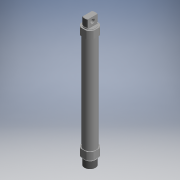
# Autodesk Inventor part: 193993 DSNU-40-300-P---(A----0-ZR)
Saved by Autodesk Inventor 2017.3 (Build 213256000, 256)
## iProperties
Part Number: 193993 DSNU-40-300-P---(A----0-ZR)
Material: Generic
Catalog Web Link: www.cadenas.de
Description: DSNU---(ZR)-Standard cylinder
Vendor: FESTO
Document SubType Name: Modeling
Designer: partserver
Manufacturer: FESTO
Mass: 189.528 g
Surface Area: 1081.04 cm^2
Volume: 189.528 cm^3
Density: 1 g/cm^3
Appearance: PSOLRGB-192-192-192
Category: PARTsolutions
Company: FESTO
Title: 193993 DSNU-40-300-P
Author: Cadenas PARTsolutions
Comments: Standard cylinder
PSOL_IDENT_0: {$CADENAS_DATA\23d-libs\festo\parts\d\dsnu\parts\dsnu_metric_zr.prj},236 {VTYP=3D},{NB=193993 DSNU-4
PSOL_IDENT_1: 0-300-P---(A----0-ZR)},{LINA=193993 DSNU-40-300-P},{NN=DSNU---(ZR)},{DATE=23.06.2020 07:36:16},{GEOM
PSOL_IDENT_2: DATE=06.03.2020 09:03:14},{VERSION=},{LINEID=80},{WBVAR=TNR,HUB,DA,PE,ZD,VS,KA,K8,KP,R8},{WBNUMERIC=
PSOL_IDENT_3: HUB,K8}  {NB=193993 DSNU-40-300-P---(A----0-ZR)},{LINA=193993 DSNU-40-300-P},{KT=DUMMY},{TNR=193993}
PSOL_IDENT_4: ,{TYP=DSNU-40},{DSNU=METRIC},{DE=D},{KDM=40},{HUB=300},{DA=P},{DA1='P','PPV','PPS'},{PE=A},{ZD=-},{V
PSOL_IDENT_5: S=-},{VSALG='-','Q'},{KA=-},{KAALG='-','S2'},{K8=0},{KP=-},{KPALG='-','KP'},{R8=-},{R81='-','R8'},{R
PSOL_IDENT_6: 8H=30.200},{A1=35},{A2=500},{A3=8},{A4=70.5},{AB=38},{AM=24},{B=38},{BB=4},{BE=M38x1,5},{BENDM=38.00
PSOL_IDENT_7: 0},{BEKDM=36.160},{BEP=1.500},{BS=9.0},{B1=54},{B2=13},{B3=38},{B4=12},{B5=32.0},{B6=14},{B7=4},{CD=
PSOL_IDENT_8: 12},{D=46},{D1=38},{D2=16},{D3=41.6},{D4=12.0},{D5=42.0},{D6=50},{D7=38},{EE=G1/4},{EENDM=13.1570},{
PSOL_IDENT_9: EEKDM=11.4450},{EW=18},{F=42},{FF=M5},{FFNDM=5.000},{FFKDM=4.019},{F1=24},{H=48},{H1=7},{KK=M12x1.25
PSOL_IDENT_10: },{KKNDM=12.0000},{KKKDM=9.8530},{KKP=1.250},{K1=M8},{K1NDM=8.000},{K1KDM=6.466},{K2=3.0},{KV=0},{KW=
PSOL_IDENT_11: 10},{L=15},{LH=15.0},{LK=18.0},{L1=153.6},{L2=84.6},{L3=12.0},{L4=30.0},{L5=27},{L6=63},{L7=33},{L8=
PSOL_IDENT_12: 25.0},{L9=29.0},{L10=104.6},{L11=116.6},{L12=77.6},{L13=162.6},{ST=9.0},{SW=13},{T=12},{WH=39},{X=3.
PSOL_IDENT_13: 3},{XC=139.6},{K1KP=56},{K2KP=M8},{K2KPNDM=8.000},{K3KP=18},{K4KP=28.0},{K5KP=89.0},{K6KP=6.8},{K7KP=
PSOL_IDENT_14: 24},{K8KP=36.0},{K9KP=17.0},{K10KP=7.0},{K11KP=20},{K12KP=G1/8},{K12KPNDM=9.728},{K13KP=69},{ZRSTART=
PSOL_IDENT_15: 55},{MHL=45.000},{ZRL=34.6},{C=21.200},{WHX=12.000},{LD1=35.800},{LD2=35.700},{AD1=14.000},{AD2=12.0
PSOL_IDENT_16: 00},{AD3=10.500},{AD4=9.000},{AD5=12.500},{MH1=11.000},{MH2=2.600},{MH3=15.200},{KP1=34.000},{KP2=30
PSOL_IDENT_17: .000},{KP3=24.000},{KP4=25.000},{KP5=45.000},{KPC=22.000},{KPF=3.000},{KPG=22.000},{KPH=83.000},{KPJ=
PSOL_IDENT_18: 23.500},{KPK=17.000},{KPL=4.500},{KPR3=1.000},{KPR=23.000},{KPS=20.500},{MLD1=55.000},{MLD2=48.000},
PSOL_IDENT_19: {MLD3=5.000},{MLL1=16.000},{PPVSTD=18.500},{PPVMH=37.000},{PPVMQ=6.500},{PPVY=10.500},{PPVZ=15.800},
PSOL_IDENT_20: {PPVA=5.000},{PPVB=0.500},{PPVC=0.800},{PPVD=1.000},{PPVE=10.000},{PPVH=16.100},{KL1=76},{SWL=6.500}
PSOL_IDENT_21: ,{K3L=8.400},{ES1=2.500},{ES2=10.500},{KPVERS=0},{HUB1=300},{NUTOFF=8.500},{DIMZJREAR=444.6},{KAVERS=
PSOL_IDENT_22: 0},{VERS=2},{H2=45}
NB: 193993 DSNU-40-300-P---(A----0-ZR)
NN: DSNU---(ZR)
NT: Standard cylinder
NBSYN: $TNR. $TYP.-$HUB1.-$DA.---($PE.$ZD.$VS.$KA.$KP.$K8.$R8.ZR)
LINA: 193993 DSNU-40-300-P
CATALOG: Festo
TNR: 193993
TYP: DSNU-40
DSNU: METRIC
DE: D
KDM: 40
HUB: 300
DA: P
DA1: 'P','PPV','PPS'
PE: A
ZD: -
VS: -
KA: -
K8: 0
KP: -
R8: -
R81: '-','R8'
R8H: 30.2
A1: 35
A2: 500
A3: 8
A4: 70.5
AB: 38
AM: 24
B: 38
BB: 4
BE: M38x1,5
BENDM: 38
BEKDM: 36.16
BEP: 1.5
BS: 9
B1: 54
B2: 13
B3: 38
B4: 12
B5: 32
B6: 14
B7: 4
CD: 12
D: 46
D1: 38
D2: 16
D3: 41.6
D4: 12
D5: 42
D6: 50
D7: 38
EE: G1/4
EENDM: 13.157
EEKDM: 11.445
EW: 18
F: 42
FF: M5
FFNDM: 5
FFKDM: 4.019
F1: 24
H: 48
H1: 7
KK: M12x1.25
KKNDM: 12
KKKDM: 9.853
KKP: 1.25
K1: M8
K1NDM: 8
K1KDM: 6.466
K2: 3
KV: 0
KW: 10
L: 15
LH: 15
LK: 18
L3: 12
L4: 30
L5: 27
L6: 63
L7: 33
L8: 25
L9: 29
L13: 162.6
ST: 9
SW: 13
T: 12
X: 3.3
K1KP: 56
K2KP: M8
K2KPNDM: 8
K3KP: 18
K4KP: 28
K5KP: 89
K6KP: 6.8
K7KP: 24
K8KP: 36
K9KP: 17
K10KP: 7
K11KP: 20
K12KP: G1/8
K12KPNDM: 9.728
K13KP: 69
MHL: 45
C: 21.2
WHX: 12
LD1: 35.8
LD2: 35.7
AD1: 14
AD2: 12
AD3: 10.5
AD4: 9
AD5: 12.5
MH1: 11
MH2: 2.6
MH3: 15.2
KP1: 34
KP2: 30
KP3: 24
KP4: 25
KP5: 45
KPC: 22
KPF: 3
KPG: 22
KPH: 83
KPJ: 23.5
KPK: 17
KPL: 4.5
KPR3: 1
KPR: 23
KPS: 20.5
MLD1: 55
MLD2: 48
MLD3: 5
MLL1: 16
PPVSTD: 18.5
PPVMH: 37
PPVMQ: 6.5
PPVY: 10.5
PPVZ: 15.8
PPVA: 5
PPVB: 0.5
PPVC: 0.8
PPVD: 1
PPVE: 10
PPVH: 16.1
SWL: 6.5
K3L: 8.4
ES1: 2.5
ES2: 10.5
NUTOFF: 8.5
H2: 45
SUPPLIER: FESTO
ARTICLENO: 193993 DSNU-40-300-P---(A----0-ZR)
BOMINFO: 193993 DSNU-40-300-P
CREATOR: CADENAS GmbH
Autodesk Inventor part; units mm, degrees
sketch "Sketch_12" plane through (0, 0, 0) normal (1, 0, 0) x (0, 1, 0)
  line L0 (0, -444.6) -> (0, 0)
  line L1 (0, 0) -> (18.08, 0)
  line L2 (18.08, 0) -> (19, -0.92)
  line L3 (19, -0.92) -> (19, -23.95)
  line L4 (19, -23.95) -> (18.0843, -24.8657)
  arc A0 (18.0843, -24.8657) -> (17.85, -25.4314) centre (18.65, -25.4314) ccw
  line L5 (17.85, -25.4314) -> (17.85, -26.2)
  arc A1 (17.85, -26.2) -> (18.65, -27) centre (18.65, -26.2) ccw
  line L6 (18.65, -27) -> (19, -27)
  line L7 (19, -27) -> (19, -30.1)
  line L8 (19, -30.1) -> (24.5, -30.1)
  line L9 (24.5, -30.1) -> (24.5, -55.05)
  line L10 (24.5, -55.05) -> (20.8, -55.05)
  line L11 (20.8, -55.05) -> (20.8, -389.55)
  line L12 (20.8, -389.55) -> (24.5, -389.55)
  line L13 (24.5, -389.55) -> (24.5, -414.5)
  line L14 (24.5, -414.5) -> (19, -414.5)
  line L15 (19, -414.5) -> (19, -417.6)
  line L16 (19, -417.6) -> (18.65, -417.6)
  arc A2 (18.65, -417.6) -> (17.85, -418.4) centre (18.65, -418.4) ccw
  line L17 (17.85, -418.4) -> (17.85, -419.1686)
  arc A3 (17.85, -419.1686) -> (18.0843, -419.7343) centre (18.65, -419.1686) ccw
  line L18 (18.0843, -419.7343) -> (19, -420.65)
  line L19 (19, -420.65) -> (19, -443.68)
  line L20 (19, -443.68) -> (18.08, -444.6)
  line L21 (18.08, -444.6) -> (0, -444.6)
  line L22 (0, -444.6) -> (0, 0)
  constraints: 46 end point, 8 point on circle, 4 centre point
revolve "Revolution1" add sketch "Sketch_12" angle 360 about axis through (0, 0, -444.6) along (0, 0, -1)
thread "Thread1" size "M38x1.5" class "6g" standard "ISO Metric profile" full length
thread "Thread2" size "M38x1.5" class "6g" standard "ISO Metric profile" full length
sketch "Sketch_1" plane through (0, 0, 0) normal (0, 0, 1) x (1, 0, 0)
  line L0 (-45, 45) -> (-45, -45)
  line L1 (-45, -45) -> (45, -45)
  line L2 (45, -45) -> (45, 45)
  line L3 (45, 45) -> (-45, 45)
  line L4 (-22.5, 22.5) -> (-22.5, -22.5)
  line L5 (-22.5, -22.5) -> (22.5, -22.5)
  line L6 (22.5, -22.5) -> (22.5, 22.5)
  line L7 (22.5, 22.5) -> (-22.5, 22.5)
  constraints: 16 end point
extrude "Extrusion1" cut sketch "Sketch_1" against normal blind 453.6
sketch "Sketch_124" plane through (0, 0, 0) normal (0, 1, 0) x (-1, 0, 0)
  line L0 (46, -415.6) -> (9, -415.6)
  line L1 (9, -415.6) -> (9, -444.6)
  line L2 (9, -444.6) -> (-9, -444.6)
  line L3 (-9, -444.6) -> (-9, -415.6)
  line L4 (-9, -415.6) -> (-46, -415.6)
  line L5 (-46, -415.6) -> (-46, -449.6)
  line L6 (-46, -449.6) -> (46, -449.6)
  line L7 (46, -449.6) -> (46, -415.6)
  constraints: 16 end point
extrude "Extrusion2" cut sketch "Sketch_124" along normal mid plane 46
sketch "Sketch_3" plane through (0, 0, -430.6) normal (0, 0, 1) x (1, 0, 0)
  line L0 (9, 0) -> (-9, 0)
  line L1 (-9, 0) -> (-9, 7.5774)
  line L2 (-9, 7.5774) -> (-8, 7)
  line L3 (-8, 7) -> (-7.5, 7)
  line L4 (-7.5, 7) -> (-7.5, 6)
  line L5 (-7.5, 6) -> (7.5, 6)
  line L6 (7.5, 6) -> (7.5, 7)
  line L7 (7.5, 7) -> (8, 7)
  line L8 (8, 7) -> (9, 7.5774)
  line L9 (9, 7.5774) -> (9, 0)
  line L10 (9, 0) -> (-9, 0)
  constraints: 22 end point
revolve "Revolution2" cut sketch "Sketch_3" angle 360 about axis through (9, 0, -430.6) along (1, 0, 0)
sketch "Sketch5" plane through (-9.6954, 22.5, -30.1) normal (0, 1, 0) x (1, 0, 0)
  point P0 (9.6954, 12)
hole "Hole1" at (0, 22.5, -42.1) direction (0, -1, 0) diameter 11.445 depth 22.5 countersink diameter 13.157 countersink angle 90 thread size "G13.157x1.337" designation "G 1/4" standard "ISO Pipe Threads"
sketch "Sketch6" plane through (-9.6954, 22.5, -389.55) normal (0, 1, 0) x (1, 0, 0)
  point P0 (9.6954, 12.95)
hole "Hole2" at (0, 22.5, -402.5) direction (0, -1, 0) diameter 11.445 depth 10.5 tip angle 120 countersink diameter 13.157 countersink angle 90 thread size "G13.157x1.337" designation "G 1/4" standard "ISO Pipe Threads"
sketch "Sketch_129" plane through (0, 0, 0) normal (1, 0, 0) x (0, 1, 0)
  line L0 (0, -377) -> (0, 9)
  line L1 (0, 9) -> (8, 9)
  line L2 (8, 9) -> (8, -67)
  line L3 (8, -67) -> (20, -67)
  line L4 (20, -67) -> (20, -377)
  line L5 (20, -377) -> (0, -377)
  line L6 (0, -377) -> (0, 9)
  constraints: 14 end point
revolve "Revolution3" cut sketch "Sketch_129" angle 360 about axis through (0, 0, -377) along (0, 0, -1)
ref_plane "FDT_FRONT_XY" through (0, 0, -30.1) normal (0, 0, -1) x (1, 0, 0)
ref_plane "FDT_FRONT_YZ" through (0, 0, -30.1) normal (1, 0, 0) x (0, -1, 0)
ref_plane "FDT_FRONT_ZX" through (0, 0, -30.1) normal (0, -1, 0) x (0, 0, -1)
ref_plane "FDT_QSFRONT_XY" through (0, 22.5, -42.1) normal (0, 1, 0) x (0, 0, 1)
ref_plane "FDT_QSFRONT_YZ" through (0, 22.5, -42.1) normal (0, 0, 1) x (1, 0, 0)
ref_plane "FDT_QSFRONT_ZX" through (0, 22.5, -42.1) normal (1, 0, 0) x (0, 1, 0)
ref_plane "FDT_QSREAR_XY" through (0, 22.5, -402.5) normal (0, 1, 0) x (0, 0, 1)
ref_plane "FDT_QSREAR_YZ" through (0, 22.5, -402.5) normal (0, 0, 1) x (1, 0, 0)
ref_plane "FDT_QSREAR_ZX" through (0, 22.5, -402.5) normal (1, 0, 0) x (0, 1, 0)
ref_plane "FDT_REAR_XY" through (0, 0, -414.5) normal (0, 0, 1) x (1, 0, 0)
ref_plane "FDT_REAR_YZ" through (0, 0, -414.5) normal (1, 0, 0) x (0, 1, 0)
ref_plane "FDT_REAR_ZX" through (0, 0, -414.5) normal (0, 1, 0) x (0, 0, 1)
ref_plane "FDT_SMBR1_XY" through (0, 0, -64.5) normal (0, 0, 1) x (-1, 0, 0)
ref_plane "FDT_SMBR1_YZ" through (0, 0, -64.5) normal (-1, 0, 0) x (0, -1, 0)
ref_plane "FDT_SMBR1_ZX" through (0, 0, -64.5) normal (0, -1, 0) x (0, 0, 1)
ref_plane "FDT_SMBR2_XY" through (0, 0, -380.1) normal (0, 0, 1) x (-1, 0, 0)
ref_plane "FDT_SMBR2_YZ" through (0, 0, -380.1) normal (-1, 0, 0) x (0, -1, 0)
ref_plane "FDT_SMBR2_ZX" through (0, 0, -380.1) normal (0, -1, 0) x (0, 0, 1)
ref_plane "FDT_SWIVELAXIS_XY" through (0, 0, -430.6) normal (1, 0, 0) x (0, 0, -1)
ref_plane "FDT_SWIVELAXIS_YZ" through (0, 0, -430.6) normal (0, 0, -1) x (0, 1, 0)
ref_plane "FDT_SWIVELAXIS_ZX" through (0, 0, -430.6) normal (0, 1, 0) x (1, 0, 0)
ref_plane "NUT_XY" through (0, 0, -8.5) normal (0, 0, -1) x (1, 0, 0)
ref_plane "NUT_YZ" through (0, 0, -8.5) normal (1, 0, 0) x (0, -1, 0)
ref_plane "NUT_ZX" through (0, 0, -8.5) normal (0, -1, 0) x (0, 0, -1)
ref_plane "ZR_XY" through (0, 0, 0) normal (0, 0, -1) x (-1, 0, 0)
ref_plane "ZR_YZ" through (0, 0, 0) normal (-1, 0, 0) x (0, 1, 0)
ref_plane "ZR_ZX" through (0, 0, 0) normal (0, 1, 0) x (0, 0, -1)
ref_plane "ZYL_XY" through (0, 0, -30.1) normal (0, 0, -1) x (1, 0, 0)
ref_plane "ZYL_YZ" through (0, 0, -30.1) normal (1, 0, 0) x (0, -1, 0)
ref_plane "ZYL_ZX" through (0, 0, -30.1) normal (0, -1, 0) x (0, 0, -1)
body "Solid1"
